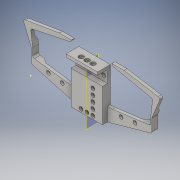
# Autodesk Inventor part: bumper_plate
Saved by Autodesk Inventor 2016 (Build 200138000, 138)
## iProperties
Created: 2016-02-15
Part Number: bumper_plate
Material: Generic
Document SubType Name: Modeling
Designer: jforce
Density: 1 g/cm^3
Appearance: Default
Author: jforce
## iProperties of the stored document bumper_plate_3DPrint.ipt
Created: 2016-02-16
Part Number: bumper_plate_3DPrint
Material: Generic
Document SubType Name: Modeling
Designer: jforce
Density: 1 g/cm^3
Appearance: Default
Author: jforce
Autodesk Inventor part; units mm, degrees
ref_plane "YZ Plane" through (0, 0, 0) normal (1, 0, 0) x (0, 1, 0)
ref_plane "XZ Plane" through (0, 0, 0) normal (0, 1, 0) x (-1, 0, 0)
ref_plane "XY Plane" through (0, 0, 0) normal (0, 0, 1) x (1, 0, 0)
sketch "Sketch1" plane through (0, 0, 0) normal (0, 0, 1) x (1, 0, 0)
  line L0 (130, 0) -> (130, 34.3878) construction
  line L1 (130, 55) -> (0, 55) construction
  line L2 (65, 55) -> (65, -3.2989) construction
  line L3 (76.7288, 0) -> (65, 0)
  line L4 (80.941, 15) -> (85.9429, 15)
  line L5 (76.7288, 0) -> (123.5984, 13.1826)
  line L6 (123.5984, 13.1826) -> (123.9312, 13.1826)
  line L7 (125.9312, 15.1826) -> (125.9312, 26.9752)
  line L8 (126.0791, 27.7299) -> (133.773, 46.6103)
  line L9 (132.245, 49.3387) -> (97.7732, 55)
  line L10 (85.5133, 55) -> (85.5133, 54.7944)
  line L11 (87.1045, 52.8366) -> (125.073, 44.9088)
  line L12 (126.6496, 42.7098) -> (124.9312, 28.567)
  line L13 (124.9312, 28.567) -> (124.9312, 21.902)
  arc A0 (126.0791, 27.7299) -> (125.9312, 26.9752) centre (127.9312, 26.9752) ccw
  arc A1 (123.9312, 13.1826) -> (125.9312, 15.1826) centre (123.9312, 15.1826) ccw
  arc A2 (123.0784, 19.9075) -> (124.9312, 21.902) centre (122.9312, 21.902) ccw
  arc A3 (85.5133, 54.7944) -> (87.1045, 52.8366) centre (87.5133, 54.7944) ccw
  line L14 (97.7732, 55) -> (85.5133, 55)
  line L15 (65, 35.1737) -> (65, 0)
  line L16 (85.9429, 15) -> (123.0784, 19.9075)
  arc A4 (133.773, 46.6103) -> (132.245, 49.3387) centre (131.9209, 47.3651) ccw
  arc A5 (126.6496, 42.7098) -> (125.073, 44.9088) centre (124.6642, 42.9511) ccw
  line L17 (65, 35.1737) -> (80.941, 35.1737)
  line L18 (80.941, 35.1737) -> (80.941, 15)
  dimension "d0" = 130
  dimension "d1" = 55
  dimension "d13" = 1
  dimension "d14" = 2
  dimension "d18" = 2
  constraints: 38 end point, 13 point on circle, 11 tangent, 6 centre point, 5 point on line, 3 equal radius, 3 horizontal, 2 parallel, 2 vertical, 1 collinear, 1 midpoint, 1 perpendicular
  measures "d0" distance of L1.end L1.start
  measures "d1" distance of L1.start L0.start
  measures "d13" distance between parallel lines of L13 L7
  measures "d14" radius of A0
  measures "d18" radius of A4
extrude "Extrusion3" add sketch "Sketch1" along normal blind 6
sketch "Sketch2" plane through (133.773, 46.6103, 6) normal (0.9260598, -0.3773768, 0) x (0, 0, -1)
  line L0 (7.8829, -18.7901) -> (3.0228, -11.0636)
  line L1 (3.0228, -11.0636) -> (3.0228, 13.8654)
  line L2 (3.0228, 13.8654) -> (7.8829, 13.8654)
  line L3 (7.8829, 13.8654) -> (7.8829, -18.7901)
  point P0 (6, -93.6468)
  constraints: 8 end point, 2 perpendicular, 1 vertical
extrude "Extrusion4" cut sketch "Sketch2" against normal through all
sketch "Sketch3" plane through (123.5984, 13.1826, 0) normal (0.2707556, -0.9626481, 0) x (0.9626481, 0.2707556, 0)
  line L0 (-1.0858, -1.1106) -> (-7.1923, 2.9772)
  line L1 (-7.1923, 2.9772) -> (-64.024, 2.9772)
  line L2 (-64.024, 2.9772) -> (-64.024, -1.1106)
  line L3 (-64.024, -1.1106) -> (-1.0858, -1.1106)
  point P0 (-122.5511, 0)
  constraints: 8 end point, 2 perpendicular, 1 horizontal
extrude "Extrusion6" cut sketch "Sketch3" against normal through all
sketch "Sketch4" plane through (85.9429, 15, 2.9772) normal (0, 0, -1) x (-1, 0, 0)
  circle A0 centre (-8.9382, -2.4263) radius 1.5 projected
  circle A1 centre (-22.9536, -0.4642) radius 1.5 projected
  point P0 (85.9429, -15)
hole "Hole1" at (108.8965, 14.5358, 2.9772) at (94.8812, 12.5737, 2.9772) direction (0, 0, 1) diameter 4 depth 3 tip angle 118 counterbore diameter 5 counterbore depth 0.85
sketch "Sketch7" plane through (0, 0, 6) normal (0, 0, 1) x (1, 0, 0)
  line L0 (65, 35.1737) -> (65, 0) projected
  line L1 (76.7288, 0) -> (123.5984, 13.1826) projected
  line L2 (65, 35.1737) -> (80.941, 35.1737)
  line L3 (80.941, 35.1737) -> (80.941, 1.1847)
  line L4 (80.941, 1.1847) -> (65, 1.1847)
  line L5 (65, 1.1847) -> (65, 35.1737)
  point P0 (0, 0)
  constraints: 8 end point, 2 parallel, 1 horizontal, 1 perpendicular, 1 point on line
extrude "Extrusion9" add sketch "Sketch7" along normal blind 5
sketch "Sketch8" plane through (80.941, 35.1737, 2.9772) normal (0, 0, -1) x (-1, 0, 0)
  line L0 (15.941, -35.1737) -> (4.2122, -35.1737) projected
  line L1 (4.2122, -35.1737) -> (0, -20.1737)
  line L2 (0, -20.1737) -> (0, 0) projected
  line L3 (0, 0) -> (15.941, 0) projected
  line L4 (15.941, 0) -> (15.941, -35.1737) projected
  line L5 (2, -2) -> (2, -19.8982)
  line L6 (2, -19.8982) -> (5.7279, -33.1737)
  line L7 (5.7279, -33.1737) -> (15.941, -33.1737)
  line L8 (15.941, -2) -> (2, -2)
  line L9 (15.941, -2) -> (15.941, -33.1737)
  line L10 (15.941, 0) -> (15.941, -33.989) projected
  point P0 (80.941, -35.1737)
  dimension "d39" = 2
  constraints: 12 end point, 2 point on line, 1 collinear, 1 other
  measures "d39" distance between parallel lines of L2 L5
extrude "Extrusion10" cut sketch "Sketch8" against normal blind 5 contours L7 L6 L5 L8 L4
ref_plane "Work Plane2" through (65, 33.1737, 5.4772) normal (-1, 0, 0) x (0, 0, 1)
mirror "Mirror2" about plane through (65, 33.1737, 5.4772) normal (-1, 0, 0)
hole "Hole3" at (71.2266, 28.3901, 7.9772) at (71.2266, 22.3901, 7.9772) at (71.2266, 16.3901, 7.9772) at (71.2266, 10.3901, 7.9772) at (71.2266, 4.3901, 7.9772) at (65.2266, 4.3901, 7.9772) at (59.2266, 4.3901, 7.9772) direction (0, 0, 1) diameter 4 depth 3 tip angle 118 counterbore diameter 5 counterbore depth 0.85
sketch "Sketch11" plane through (80.941, 35.1737, 11) normal (0, 1, 0) x (1, 0, 0)
  line L0 (-31.8821, 5) -> (0, 5) projected
  line L1 (-31.8821, 8.0228) -> (-31.8821, 5) projected
  line L2 (0, 5) -> (-31.8821, 5)
  line L3 (-31.8821, 5) -> (-31.8821, 8.0228)
  line L4 (-31.8821, 8.0228) -> (0, 8.0228)
  line L5 (0, 8.0228) -> (0, 5)
  point P0 (-80.941, 11)
  constraints: 8 end point, 2 parallel, 1 horizontal, 1 perpendicular
extrude "Extrusion11" add sketch "Sketch11" along normal blind 15
sketch "Sketch12" plane through (85.9429, 15, 2.9772) normal (0, 0, -1) x (-1, 0, 0)
  point P0 (85.9429, -15)
sketch "Sketch13" plane through (49.059, 35.1737, 6) normal (0, 0, 1) x (1, 0, 0)
  line L0 (0, -20.1737) -> (0, 15) projected
  line L1 (31.8821, -20.1737) -> (31.8821, 15) projected
  line L2 (0, 15) -> (31.8821, 15)
  line L3 (31.8821, 15) -> (31.8821, 12)
  line L4 (31.8821, 12) -> (0, 12)
  line L5 (0, 12) -> (0, 15)
  point P0 (-49.059, -35.1737)
  dimension "d58" = 3
  constraints: 8 end point, 2 parallel, 1 horizontal, 1 perpendicular, 1 point on line
  measures "d58" distance of L2.end L3.end
extrude "Extrusion12" add sketch "Sketch13" along normal blind 10
sketch "Sketch14" plane through (80.941, 50.1737, 11) normal (0, 1, 0) x (1, 0, 0)
  line L0 (-7.7524, 0) -> (-11.6765, 0) projected
  line L1 (0, 0) -> (-31.8821, 0) projected
  point P0 (-80.941, 11)
  point P1 (-9.5459, 0)
  constraints: 1 point on line
hole "Hole4" at (71.3951, 50.1737, 11) direction (0, -1, 0) diameter 4 depth 3 tip angle 118 counterbore diameter 5 counterbore depth 0.85
pattern_linear "Rectangular Pattern1" count 3 spacing 6 along (-1, 0, 0) of "Hole4"
sketch "Sketch15" plane through (85.9429, 15, 2.9772) normal (0, 0, -1) x (-1, 0, 0)
  circle A0 centre (8.7164, 19.3901) radius 2 projected
  point P0 (85.9429, -15)
sketch "Sketch16" plane through (85.9429, 15, 2.9772) normal (0, 0, -1) x (-1, 0, 0)
  circle A0 centre (8.7164, 25.3901) radius 2 projected
  point P0 (85.9429, -15)
hole "Hole5" at (77.2266, 40.3901, 2.9772) direction (0, 0, 1) diameter 4 depth 3 tip angle 118 counterbore diameter 5 counterbore depth 0.85
pattern_linear "Rectangular Pattern2" count 5 spacing 6 along (-1, 0, 0) of "Hole5"
body "Solid3"
